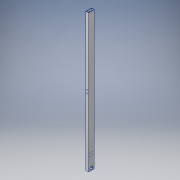
# Autodesk Inventor part: main beam
Saved by Autodesk Inventor 2017 (Build 210142000, 142)
## iProperties
Created: 2017-12-26
Part Number: main beam
Material: Aluminum 6061
Document SubType Name: Modeling
Designer: Micah
Density: 2.7 g/cm^3
Appearance: Aluminum - Flat
Mass: 1453.23 g
Surface Area: 3405.97 cm^2
Volume: 538.234 cm^3
Author: Micah
Autodesk Inventor part; units mm, degrees
ref_plane "YZ Plane" through (0, 0, 0) normal (1, 0, 0) x (0, 1, 0)
ref_plane "XZ Plane" through (0, 0, 0) normal (0, 1, 0) x (-1, 0, 0)
ref_plane "XY Plane" through (0, 0, 0) normal (0, 0, 1) x (1, 0, 0)
sketch "Sketch2" plane through (0, 0, 0) normal (0, 1, 0) x (-1, 0, 0)
  line L0 (0, 0) -> (-25.4, 0)
  line L1 (-25.4, 0) -> (0, 0)
  line L2 (0, 0) -> (0, -50.8)
  line L3 (0, -50.8) -> (-25.4, -50.8)
  line L4 (-25.4, -50.8) -> (-25.4, 0)
  line L5 (-22.225, -47.625) -> (-3.175, -47.625)
  line L6 (-3.175, -47.625) -> (-3.175, -3.175)
  line L7 (-3.175, -3.175) -> (-22.225, -3.175)
  line L8 (-22.225, -3.175) -> (-22.225, -47.625)
  dimension "d2" = 25.4
  dimension "d3" = 50.8
  dimension "d4" = 19.05
  dimension "d5" = 44.45
  dimension "d6" = 3.175
  dimension "d7" = 3.175
  constraints: 18 end point, 4 parallel, 2 horizontal, 2 perpendicular
  measures "d2" distance of L2.end L3.end
  measures "d3" distance of L1.end L2.end
  measures "d4" distance of L7.end L6.end
  measures "d5" distance of L6.end L5.end
  measures "d6" distance between parallel lines of L4 L8
  measures "d7" distance between parallel lines of L5 L3
extrude "Extrusion1" add sketch "Sketch2" along normal blind 1219.2
sketch "Sketch3" plane through (25.4, 0, -50.8) normal (0, 0, -1) x (-1, 0, 0)
  line L0 (25.4, 1219.2) -> (25.4, 609.6) construction
  line L1 (25.4, 0) -> (25.4, 1219.2) projected
  line L2 (25.4, 609.6) -> (0, 609.6) construction
  line L3 (0, 0) -> (0, 1219.2) projected
  line L4 (12.7, 609.6) -> (12.7, 622.3) construction
  circle A0 centre (12.7, 622.3) radius 3.175
  line L5 (12.7, 609.6) -> (12.7, 596.9) construction
  circle A1 centre (12.7, 596.9) radius 3.175
  dimension "d10" = 1219.2
  dimension "d11" = 609.6
  dimension "d12" = 12.7
  dimension "d13" = 6.35
  constraints: 8 end point, 3 midpoint, 2 centre point, 2 coincident, 2 symmetric about line, 1 vertical, 1 other
  measures "d10" distance of L1.start L0.start
  measures "d11" distance of L0.start L0.end
  measures "d12" distance of L4.start L4.end
  measures "d13" diameter of A0
extrude "Extrusion2" cut sketch "Sketch3" against normal blind 1219.2
sketch "Sketch4" plane through (0, 0, -50.8) normal (-1, 0, 0) x (0, 0, 1)
  line L0 (3.175, 1219.2) -> (47.625, 1219.2) projected
  line L1 (25.4, 1219.2) -> (25.4, 1190.625)
  circle A0 centre (25.4, 1190.625) radius 14.2875
  point P0 (50.8, 0)
  dimension "d16" = 28.575
  dimension "d17" = 28.575
  constraints: 2 end point, 1 centre point, 1 coincident, 1 midpoint, 1 vertical
  measures "d16" distance of L1.start L1.end
  measures "d17" diameter of A0
extrude "Extrusion3" cut sketch "Sketch4" against normal blind 6.35
sketch "Sketch5" plane through (25.4, 0, 0) normal (1, 0, 0) x (0, 0, -1)
  line L0 (47.625, 0) -> (3.175, 0) construction
  line L1 (25.4, 0) -> (25.4, 114.3) construction
  line L2 (50.8, 0) -> (50.8, 1219.2) construction
  line L3 (50.8, 0) -> (38.1, 0) construction
  circle A0 centre (38.1, 114.3) radius 1.5875
  circle A1 centre (12.7, 114.3) radius 1.5875
  line L4 (0, 0) -> (0, 1219.2) construction
  line L5 (0, 127) -> (50.8, 127) construction
  circle A2 centre (38.1, 139.7) radius 1.5875
  circle A3 centre (12.7, 139.7) radius 1.5875
  dimension "d20" = 114.3
  dimension "d21" = 12.7
  dimension "d22" = 3.175
  constraints: 6 end point, 4 centre point, 3 point on line, 3 symmetric about line, 1 midpoint, 1 perpendicular, 1 vertical, 3 other
  measures "d20" distance of L1.start L1.end
  measures "d21" distance of L2.start L3.end
  measures "d22" diameter of A0
hole "Hole1" at (25.4, 139.7, -12.7) at (25.4, 114.3, -12.7) at (25.4, 114.3, -38.1) at (25.4, 139.7, -38.1) direction (-1, 0, 0) diameter 3.175 depth 3.175 tip angle 118
sketch "Sketch6" plane through (25.4, 0, 0) normal (1, 0, 0) x (0, 0, -1)
  line L0 (11.1125, 0) -> (11.1125, 22.815)
  line L1 (50.8, 0) -> (0, 0) projected
  line L2 (39.6875, 0) -> (39.6875, 22.815)
  line L3 (0, 0) -> (0, 1219.2) projected
  line L4 (50.8, 0) -> (50.8, 1219.2) projected
  circle A0 centre (25.4, 19.05) radius 14.7752
  dimension "d31" = 11.1125
  dimension "d32" = 11.1125
  dimension "d33" = 19.05
  constraints: 4 end point, 2 vertical, 1 point on line, 3 other
  measures "d31" distance between parallel lines of L3 L0
  measures "d32" distance between parallel lines of L4 L2
  measures "d33" distance from line of L1 point (25.4, 19.05)
hole "Hole2" at (25.4, 19.05, -25.4) direction (-1, 0, 0) diameter 28.575 depth 3.175 tip angle 118
body "Solid1"
